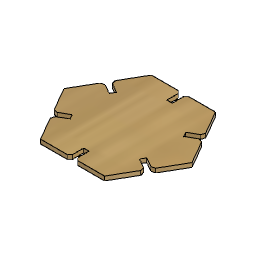
Parametric_hexagon (Autodesk Fusion 360 design; units mm, degrees)
Autodesk Fusion 360 part; units mm, degrees
sketch "Sketch1" plane through (0, 0, 0) normal (0, 0, 1) x (1, 0, 0) in component "Component"
  line L0 (-4.9635, 8.6391) -> (5.0365, 8.6391)
  line L1 (-9.9634, 0.021) -> (-4.9634, 8.6813)
  line L2 (-4.9999, -8.6181) -> (-9.9999, 0.0422)
  line L3 (4.9635, -8.6391) -> (-5.0365, -8.6391)
  line L4 (9.9634, -0.021) -> (4.9634, -8.6813)
  line L5 (4.9999, 8.6181) -> (9.9999, -0.0422)
  dimension "d2" = 10
  dimension "d4" = 360
  dimension "d5" = 10
  dimension "d6" = 10
  constraint horizontal L0
  measures "d2" distance of L0.start L0.end
  measures "d5" distance of origin L0.end
  measures "d6" distance of origin L1.end
sketch "Sketch2" plane through (0, 0, 0) normal (0, 0, 1) x (1, 0, 0) in component "Component"
  line L0 (23.094, 40) -> (0, 0) construction
  line L1 (0, 0) -> (-23.094, 40) construction
  line L2 (1.925, 38) -> (1.925, 30)
  line L3 (1.925, 30) -> (-1.925, 30)
  line L4 (-1.925, 30) -> (-1.925, 38)
  line L5 (-23.094, 40) -> (-3.925, 40)
  line L6 (3.925, 40) -> (23.094, 40)
  line L7 (-3.925, 40) -> (-1.925, 38)
  line L8 (0, 30) -> (0, 40) construction
  line L9 (3.925, 40) -> (1.925, 38)
  line L10 (-32.6785, 23.3991) -> (-23.094, 40)
  line L11 (-32.6785, 23.3991) -> (-31.9465, 20.6671)
  line L12 (-26.9433, 13.3329) -> (-33.8715, 17.3329)
  line L13 (-25.9808, 15) -> (-34.641, 20) construction
  line L14 (-36.6035, 16.6009) -> (-33.8715, 17.3329)
  line L15 (-46.188, 0) -> (-36.6035, 16.6009)
  line L16 (-25.0183, 16.6671) -> (-26.9433, 13.3329)
  line L17 (-31.9465, 20.6671) -> (-25.0183, 16.6671)
  line L18 (-36.6035, -16.6009) -> (-46.188, 0)
  line L19 (-36.6035, -16.6009) -> (-33.8715, -17.3329)
  line L20 (-25.0183, -16.6671) -> (-31.9465, -20.6671)
  line L21 (-25.9808, -15) -> (-34.641, -20) construction
  line L22 (-32.6785, -23.3991) -> (-31.9465, -20.6671)
  line L23 (-23.094, -40) -> (-32.6785, -23.3991)
  line L24 (-26.9433, -13.3329) -> (-25.0183, -16.6671)
  line L25 (-33.8715, -17.3329) -> (-26.9433, -13.3329)
  line L26 (-3.925, -40) -> (-23.094, -40)
  line L27 (-3.925, -40) -> (-1.925, -38)
  line L28 (1.925, -30) -> (1.925, -38)
  line L29 (0, -30) -> (0, -40) construction
  line L30 (3.925, -40) -> (1.925, -38)
  line L31 (23.094, -40) -> (3.925, -40)
  line L32 (-1.925, -30) -> (1.925, -30)
  line L33 (-1.925, -38) -> (-1.925, -30)
  line L34 (32.6785, -23.3991) -> (23.094, -40)
  line L35 (32.6785, -23.3991) -> (31.9465, -20.6671)
  line L36 (26.9433, -13.3329) -> (33.8715, -17.3329)
  line L37 (25.9808, -15) -> (34.641, -20) construction
  line L38 (36.6035, -16.6009) -> (33.8715, -17.3329)
  line L39 (46.188, 0) -> (36.6035, -16.6009)
  line L40 (25.0183, -16.6671) -> (26.9433, -13.3329)
  line L41 (31.9465, -20.6671) -> (25.0183, -16.6671)
  line L42 (36.6035, 16.6009) -> (46.188, 0)
  line L43 (36.6035, 16.6009) -> (33.8715, 17.3329)
  line L44 (25.0183, 16.6671) -> (31.9465, 20.6671)
  line L45 (25.9808, 15) -> (34.641, 20) construction
  line L46 (32.6785, 23.3991) -> (31.9465, 20.6671)
  line L47 (23.094, 40) -> (32.6785, 23.3991)
  line L48 (26.9433, 13.3329) -> (25.0183, 16.6671)
  line L49 (33.8715, 17.3329) -> (26.9433, 13.3329)
  point P0 (0, 40)
  point P1 (0, 40)
  point P2 (-34.641, 20)
  point P3 (-34.641, 20)
  point P4 (-34.641, -20)
  point P5 (-34.641, -20)
  point P6 (0, -40)
  point P7 (0, -40)
  point P8 (34.641, -20)
  point P9 (34.641, -20)
  point P10 (34.641, 20)
  point P11 (34.641, 20)
  dimension "d8" = 40
  dimension "d10" = 60
  dimension "d22" = 45
  dimension "d23" = 2
  dimension "d24" = 3.85
  dimension "d25" = 10
  dimension "d27" = 360
  constraint horizontal L5
  constraint coincident L0.end L1.start
  constraint equal L0 L1
  constraint vertical L2
  constraint horizontal L3
  constraint vertical L4
  constraint coincident P1 P0
  constraint collinear L5 L6
  constraint coincident P1 L5
  constraint midpoint L3 L8.start
  constraint perpendicular L3 L8
  constraint symmetric L5.end L8 L6.start
  constraint symmetric L4.end L8 L2.start
  constraint equal L5 L6
  measures "d8" distance of L0.end L5
  measures "d10" angle of L0 L1
  measures "d22" angle of L5 L7
  measures "d23" horizontal distance of L5.end L4.end
  measures "d24" distance of L2.end L3.end
  measures "d25" vertical distance of L2.end L6.start
extrude "Extrude1" add sketch "Sketch2" along normal blind 3
component "Component" placed x (1, 0, 0) y (0, 1, 0) z (0, 0, 1) at (0, 0, 0)
equation "Radius = 40 mm"
equation "d8 = Radius"
equation "NumberSides = 6"
equation "d10 = Angle"
equation "Angle = ( 360 / NumberSides ) * 1 deg"
equation "Thickness = 4 mm"
equation "Kerf = 0.15 mm"
equation "Slot = 10 mm"
equation "Chamfer_Angle = 45 deg"
equation "Chamfer_Size = 2 mm"
equation "d22 = Chamfer_Angle"
equation "d23 = Chamfer_Size"
equation "d24 = Thickness - Kerf"
equation "d25 = Slot"
equation "d26 = NumberSides"
